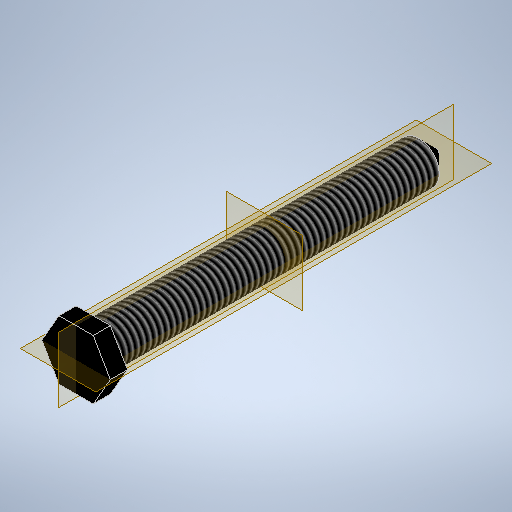
# Autodesk Inventor part: Sessao9__08_04_2025_0002_001
Saved by Autodesk Inventor 2025.2 (Build 292293000, 293)
## iProperties
Created: 2025-04-08
Part Number: Sessao9__08_04_2025_0002_001
Material: Ouro
Document SubType Name: Modeling
Designer: Gustavo Sousa
Density: 19.3 g/cm^3
Appearance: Anodizado - Preto
Author: Gustavo Sousa
Autodesk Inventor part; units mm, degrees
sketch "Esboço1" plane through (0, 0, 0) normal (0, 0, 1) x (1, 0, 0)
  circle A0 centre (0, 0) radius 6
  dimension "d0" = 12
  constraints: 1 centre point, 1 coincident
  measures "d0" diameter of A0
extrude "Extrusão1" add sketch "Esboço1" along normal mid plane 100
sketch "Esboço2" plane through (0, 0, 50) normal (0, 0, 1) x (1, 0, 0)
  line L0 (5, 8.6603) -> (10, 0)
  line L1 (10, 0) -> (5, -8.6603)
  line L2 (5, -8.6603) -> (-5, -8.6603)
  line L3 (-5, -8.6603) -> (-10, 0)
  line L4 (-10, 0) -> (-5, 8.6603)
  line L5 (-5, 8.6603) -> (5, 8.6603)
  point P0 (0, 0)
  point P1 (0, 0)
  dimension "d3" = 10
  constraints: 12 end point, 1 coincident, 1 horizontal, 13 other
  measures "d3" distance of L4.end L0.start
extrude "Extrusão2" add sketch "Esboço2" along normal blind 5
thread "Rosca1" size "M12x1.75" class "6g" standard "ANSI Metric M Profile" length 100
chamfer "Chanfro1" distance 2 angle 45 1 edges at (-6, 0, 50)
chamfer "Chanfro2" distance 5 angle 45 1 edges at (-6, 0, -50)
